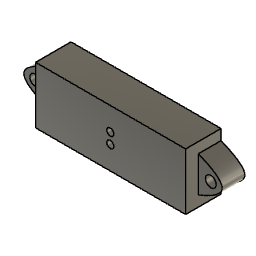
L Distance Sensor Mount (Autodesk Fusion 360 archive; units mm, degrees)
design "Distance Sensor"
Autodesk Fusion 360 part; units mm, degrees
sketch "Sketch2" plane through (0, 0, 0) normal (0, 1, 0) x (1, 0, 0)
  line L0 (0, 0) -> (42.015, 0)
  line L1 (42.015, 0) -> (42.015, -15.89)
  line L2 (42.015, -15.89) -> (0, -15.89)
  line L3 (0, -15.89) -> (0, 0)
  circle A0 centre (45.515, -7.945) radius 1.5
  line L4 (42.015, -7.945) -> (48.69, -7.945)
  spline S0 degree 5 poles (42.015, -12.945) (42.5156, -12.7419) (43.4745, -12.3366) (44.7863, -11.7309) (46.2763, -10.9278) (47.6689, -9.93) (48.5399, -8.9364) (48.8392, -7.945) (48.5399, -6.9536) (47.6689, -5.96) (46.2763, -4.9622) (44.7863, -4.1591) (43.4745, -3.5534) (42.5156, -3.1481) (42.015, -2.945) knots 0 0 0 0 0 0 0.1 0.2 0.3 0.4 0.5 0.6 0.7 0.8 0.9 1 1 1 1 1 1
  line L5 (20.92, -15.89) -> (20.92, 0)
  spline S1 degree 5 poles (-0.175, -12.945) (-0.6756, -12.7419) (-1.6345, -12.3366) (-2.9463, -11.7309) (-4.4363, -10.9278) (-5.8289, -9.93) (-6.6999, -8.9364) (-6.9992, -7.945) (-6.6999, -6.9536) (-5.8289, -5.96) (-4.4363, -4.9622) (-2.9463, -4.1591) (-1.6345, -3.5534) (-0.6756, -3.1481) (-0.175, -2.945) knots 0 0 0 0 0 0 0.1 0.2 0.3 0.4 0.5 0.6 0.7 0.8 0.9 1 1 1 1 1 1
  line L6 (40.2192, -13.6735) -> (43.8108, -12.2165)
  line L7 (43.8108, -3.6735) -> (40.2192, -2.2165)
  line L8 (1.6208, -13.6735) -> (-1.9708, -12.2165)
  line L9 (-1.9708, -3.6735) -> (1.6208, -2.2165)
  circle A1 centre (-3.675, -7.945) radius 1.5
  line L10 (-0.175, -7.945) -> (-6.85, -7.945)
  circle A2 centre (20.92, -9.45) radius 1
  circle A3 centre (20.92, -6.45) radius 1
  line L11 (-0.175, -12.945) -> (0, -13.016)
  line L12 (-0.175, -7.945) -> (0, -7.945)
  line L13 (-0.175, -2.945) -> (0, -2.874)
  dimension "d2" = 15.89
  dimension "d3" = 3
  dimension "d5" = 3.5
  dimension "d6" = 10
  dimension "d7" = 2.945
  dimension "d8" = 15.89
  dimension "d19" = 2
  dimension "d20" = 2
  dimension "d21" = 3
  dimension "d22" = 6.45
  dimension "d25" = 49.19
  dimension "d26" = 42.19
  dimension "d27" = 55.54
  dimension "d29" = 7.945
  constraint horizontal L0
  constraint vertical L1
  constraint horizontal L2
  constraint vertical L3
  constraint coincident L0.start L3.end
  constraint midpoint L1 L4.start
  constraint perpendicular L1 L4
  constraint coincident L1 S0.start
  constraint coincident L1 S0.end
  constraint coincident L2 L5.start
  constraint coincident L0 L5.end
  constraint perpendicular L0 L5
  constraint midpoint S0.start L6
  constraint midpoint S0.end L7
  constraint symmetric A0 L5 A1
  constraint symmetric L4.start L5 L10.start
  constraint symmetric L4.end L5 L10.end
  constraint symmetric S0.start L5 S1.start
  constraint symmetric S0.end L5 S1.end
  constraint symmetric L5 L6.start L8.start
  constraint symmetric L5 L6.end L8.end
  constraint symmetric L5 L7.start L9.start
  constraint symmetric L5 L7.end L9.end
  constraint coincident L5 A2.centre
  constraint coincident L5 A3.centre
  constraint coincident L8 L11.end
  constraint coincident L3 L11.end
  constraint midpoint L3 L12.end
  constraint perpendicular L3 L12
  constraint coincident L9 L13.end
  constraint coincident L3 L13.end
  measures "d2" distance of L0.start L2.end
  measures "d3" diameter of A0
  measures "d5" distance of L1 A0.centre
  measures "d6" distance of S0.start S0.end
  measures "d7" distance of L2 S0.start
  measures "d8" distance of L0.end L1.end
  measures "d19" diameter of A2
  measures "d20" diameter of A3
  measures "d21" distance of A2.centre A3.centre
  measures "d22" distance of L0 A3.centre
  measures "d25" distance of A0.centre A1.centre
  measures "d26" distance of L4.start L10.start
  measures "d27" distance of L4.end L10.end
  measures "d29" distance of L0 A1.centre
extrude "Extrude1" add sketch "Sketch2" along normal blind 6.35 contours L0 L2 L3 L5 A2 A3 | L0 L1 L2 L5 A2 A3 | L3 S1 L9 A1 L10 L12 L13 | L5 A3 | L5 A3 | L3 S1 L8 A1 L10 L11 L12 | L1 A0 L4 S0 | L1 A0 L4 S0 | L5 A2 | L5 A2
extrude "Extrude2" add sketch "Sketch2" against normal blind 3.56 contours L0 L2 L3 L5 A2 A3 | L0 L1 L2 L5 A2 A3 | L5 A3 | L5 A3 | L5 A2 | L5 A2
extrude "Extrude3" cut sketch "Sketch2" against normal blind 25 contours L5 A3 | L5 A3 | L5 A2 | L5 A2
equation "d4 = 6.5 mm"
equation "d5 = d4 - 1.5 mm - d3 / 2"
equation "d7 = ( d8 - d6 ) / 2"
equation "d12 = -9.91 mm + 6.35 mm"
equation "d29 = d2 / 2"

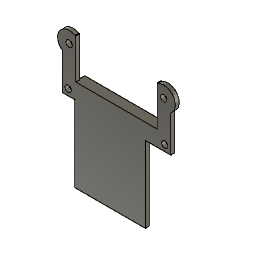
design "hingeMount"
Autodesk Fusion 360 part; units mm, degrees
sketch "Sketch1" plane through (0, 0, 0) normal (0, 0, 1) x (1, 0, 0)
  circle A0 centre (0, 0) radius 1.6
  circle A1 centre (0, 0) radius 3.1
  line L0 (-2.192, 2.192) -> (-8.6341, -4.25)
  line L1 (-2.192, 2.192) -> (4.2881, 2.192) construction
  line L2 (2.192, 2.192) -> (8.6341, -4.25)
  line L3 (2.192, 2.192) -> (10.3664, 2.192) construction
  line L4 (-8.6341, -4.25) -> (8.6341, -4.25)
  dimension "d1" = 3.2
  dimension "d2" = 1.5
  dimension "d3" = 135
  dimension "d4" = 45
  dimension "d5" = 4.25
  constraint coincident A0.centre A1.centre
  constraint horizontal L1
  constraint coincident A1 L0.start
  constraint tangent A1 L0
  constraint horizontal L3
  constraint coincident A1 L2.start
  constraint tangent A1 L2
  constraint horizontal L4
  measures "d1" diameter of A0
  measures "d3" angle of L0 L1
  measures "d4" angle of L2 L3
  measures "d5" distance of A0.centre L4
extrude "Extrude1" add sketch "Sketch1" along normal blind 12.5
extrude "Extrude2" add 1 faces at (-2.878, -4.25, 4.1667) along direction (0, -1, 0) blind 0.8
sketch "Sketch2" plane through (0, -5.05, 0) normal (0, -1, 0) x (1, 0, 0)
  line L0 (-8.6341, 0) -> (8.6341, 0)
  line L1 (8.6341, 0) -> (8.6341, 12.5)
  line L2 (8.6341, 12.5) -> (-8.6341, 12.5)
  line L3 (-8.6341, 12.5) -> (-8.6341, 0)
  line L4 (-8.6341, 12.5) -> (8.6341, 12.5)
  line L5 (8.6341, 12.5) -> (8.6341, -2.5)
  line L6 (8.6341, -2.5) -> (-8.6341, -2.5)
  line L7 (-8.6341, -2.5) -> (-8.6341, 12.5)
  line L8 (-8.6341, 12.5) -> (8.6341, 12.5)
  line L9 (8.6341, 12.5) -> (8.6341, 14)
  line L10 (8.6341, 14) -> (-8.6341, 14)
  line L11 (-8.6341, 14) -> (-8.6341, 12.5)
  dimension "d10" = 15
  dimension "d11" = 1.5
  constraint horizontal L4
  constraint vertical L5
  constraint horizontal L6
  constraint vertical L7
  constraint coincident L2.end L3.start
  constraint horizontal L8
  constraint vertical L9
  constraint horizontal L10
  constraint vertical L11
  measures "d10" distance of L2.end L6.end
  measures "d11" distance of L2.end L10.end
extrude "Extrude3" add sketch "Sketch2" along normal blind 1.5
sketch "Sketch3" plane through (0, -6.55, 0) normal (0, -1, 0) x (1, 0, 0)
  line L0 (8.6341, -2.5) -> (8.6341, 14)
  line L1 (8.6341, 14) -> (-8.6341, 14)
  line L2 (-8.6341, 14) -> (-8.6341, -2.5)
  line L3 (-8.6341, -2.5) -> (8.6341, -2.5)
  line L4 (-21, -2.5) -> (21, -2.5)
  line L5 (21, -2.5) -> (21, 64)
  line L6 (21, 64) -> (-21, 64)
  line L7 (-21, 64) -> (-21, -2.5)
  dimension "d14" = 42
  dimension "d15" = 50
  constraint horizontal L4
  constraint vertical L5
  constraint horizontal L6
  constraint vertical L7
  constraint midpoint L3 L4
  measures "d14" distance of L4.start L4.end
  measures "d15" distance of L1 L6
extrude "Extrude4" add sketch "Sketch3" along normal blind 2
extrude "Extrude5" add 1 faces at (2.878, -5.55, 14) along direction (0, 0, 1) blind 27
sketch "Sketch4" plane through (0, -6.55, 0) normal (0, 1, 0) x (-1, 0, 0)
  line L0 (8.6341, -2.5) -> (21, -2.5)
  line L1 (21, -2.5) -> (21, 64)
  line L2 (21, 64) -> (-21, 64)
  line L3 (-21, 64) -> (-21, -2.5)
  line L4 (-23.9, 59) -> (23.9, 59)
  circle A0 centre (-23.9, 59) radius 5.7801
  circle A1 centre (23.9, 59) radius 5.7801
  line L5 (-23.9, 53.2199) -> (-21, 53.2199)
  line L6 (-21, 53.2199) -> (-21, 40.8199)
  line L7 (-21, 40.8199) -> (-23.9, 40.8199)
  line L8 (-23.9, 40.8199) -> (-23.9, 53.2199)
  line L9 (-23.9, 40.8199) -> (-27.4, 40.8199)
  line L10 (-27.4, 40.8199) -> (-27.4, 53.2199)
  line L11 (-27.4, 53.2199) -> (-23.9, 53.2199)
  line L12 (-23.9, 53.2199) -> (-23.9, 40.8199)
  line L13 (-27.4, 53.2199) -> (-27.4, 54.4)
  line L14 (21, 40.8199) -> (27.4, 40.8199)
  line L15 (27.4, 40.8199) -> (27.4, 53.2199)
  line L16 (27.4, 53.2199) -> (21, 53.2199)
  line L17 (21, 53.2199) -> (21, 40.8199)
  line L18 (27.4, 53.2199) -> (27.4, 54.4)
  line L19 (-27.4, 40.8199) -> (-21, 40.8199)
  line L20 (-21, 40.8199) -> (-21, 35.8199)
  line L21 (-21, 35.8199) -> (-27.4, 35.8199)
  line L22 (-27.4, 35.8199) -> (-27.4, 40.8199)
  line L23 (21, 40.8199) -> (27.4, 40.8199)
  line L24 (27.4, 40.8199) -> (27.4, 35.8199)
  line L25 (27.4, 35.8199) -> (21, 35.8199)
  line L26 (21, 35.8199) -> (21, 40.8199)
  circle A2 centre (-23.9, 59) radius 1.6
  circle A3 centre (23.9, 59) radius 1.6
  line L27 (-27.4, 40.8199) -> (27.4, 40.8199)
  line L28 (27.4, 40.8199) -> (27.4, 43.8699)
  line L29 (27.4, 43.8699) -> (-27.4, 43.8699)
  line L30 (-27.4, 43.8699) -> (-27.4, 40.8199)
  line L31 (-8.6341, 41) -> (8.6341, 41)
  line L32 (8.6341, 41) -> (8.6341, -2.5)
  line L33 (-21, -2.5) -> (-8.6341, -2.5)
  line L34 (-8.6341, -2.5) -> (-8.6341, 41)
  point P0 (0, 59)
  point P1 (-23.9, 53.2199)
  dimension "d21" = 47.8
  dimension "d22" = 5
  dimension "d23" = 21
  dimension "d26" = 12.4
  dimension "d27" = 2.9
  dimension "d28" = 3.5
  dimension "d29" = 6.4
  dimension "d31" = 12.4
  dimension "d32" = 5
  dimension "d33" = 5
  dimension "d34" = 3.2
  dimension "d35" = 3.2
  dimension "d36" = 3.05
  constraint horizontal L4
  constraint midpoint L4 P0
  constraint coincident L4.start A0.centre
  constraint coincident L2.end A0
  constraint coincident L4.end A1.centre
  constraint coincident L1.end A1
  constraint coincident A0 P1
  constraint horizontal L5
  constraint vertical L6
  constraint horizontal L7
  constraint vertical L8
  constraint coincident L3 L6.end
  constraint coincident P1 L5.start
  constraint horizontal L9
  constraint vertical L10
  constraint horizontal L11
  constraint vertical L12
  constraint coincident A0 L13.end
  constraint perpendicular L11 L13
  constraint horizontal L14
  constraint vertical L15
  constraint horizontal L16
  constraint vertical L17
  constraint coincident L1 L14.start
  constraint coincident A1 L18.end
  constraint perpendicular L16 L18
  constraint tangent A1 L16
  constraint horizontal L19
  constraint vertical L20
  constraint horizontal L21
  constraint vertical L22
  constraint horizontal L23
  constraint vertical L24
  constraint horizontal L25
  constraint vertical L26
  constraint coincident L14.end L15.start
  constraint concentric A0 A2
  constraint concentric A1 A3
  constraint horizontal L27
  constraint vertical L28
  constraint horizontal L29
  constraint vertical L30
  constraint coincident L15 L28.end
  measures "d21" distance of L4.start L4.end
  measures "d22" distance of L2 L4
  measures "d23" distance of L3 P0
  measures "d26" distance of P1 L7.end
  measures "d27" distance of L6.end L7.end
  measures "d28" distance of L7.end L9.end
  measures "d29" distance of L14.start L14.end
  measures "d31" distance of L14.end L15.end
  measures "d32" distance of L9.end L21.end
  measures "d33" distance of L14.start L25.end
  measures "d34" diameter of A2
  measures "d35" diameter of A3
  measures "d36" distance of L9.end L29.end
extrude "Extrude6" add sketch "Sketch4" against normal blind 2 contours L1 L14 L23 L24 L25 L26 L27 | L1 L14 L15 L17 L23 L27 L28 L29 | L3 L6 L7 L8 L12 L19 L27 L29 | L3 L7 L9 L19 L20 L21 L22 L27 | L1 L15 L16 L17 L29 | L3 L5 L6 L8 L12 L29 | L8 L9 L10 L12 L19 L27 L29 L30 | L1 A1 L16 | L3 A0 L5 | L8 L10 L11 L12 L29 | L1 A1 | A1 L16 L18 | L3 A0 | A0 L11 L13
extrude "Extrude7" add sketch "Sketch4" along normal blind 3 contours L1 L3 L6 L17 L27 L29 L31 L32 L34 | L27 L31 L32 L34
chamfer "Chamfer1" distance 1.5 angle 45 4 edges at (-14.817, -6.55, 40.8199) (-8.6341, -6.55, 19.1599) (8.6341, -6.55, 19.1599) (14.817, -6.55, 40.8199)
sketch "Sketch5" plane through (0, -6.55, 0) normal (0, 1, 0) x (-1, 0, 0)
  line L0 (10.1341, 39.3199) -> (10.1341, -2.5)
  line L1 (10.1341, -2.5) -> (21, -2.5)
  line L2 (21, -2.5) -> (21, 35.8199)
  line L3 (21, 35.8199) -> (27.4, 35.8199)
  line L4 (27.4, 35.8199) -> (27.4, 54.4)
  arc A0 (27.4, 54.4) -> (21, 64) centre (23.9, 59) ccw
  line L5 (21, 64) -> (-21, 64)
  arc A1 (-21, 64) -> (-27.4, 54.4) centre (-23.9, 59) ccw
  line L6 (-27.4, 54.4) -> (-27.4, 35.8199)
  line L7 (-27.4, 35.8199) -> (-21, 35.8199)
  line L8 (-21, 35.8199) -> (-21, -2.5)
  line L9 (-21, -2.5) -> (-10.1341, -2.5)
  line L10 (-10.1341, -2.5) -> (-10.1341, 39.3199)
  line L11 (-10.1341, 39.3199) -> (-21, 39.3199)
  line L12 (-21, 43.8699) -> (21, 43.8699)
  line L13 (21, 39.3199) -> (10.1341, 39.3199)
  circle A2 centre (23.9, 59) radius 1.6
  circle A3 centre (-23.9, 59) radius 1.6
  line L14 (-21, 43.8699) -> (21, 43.8699)
  line L15 (-20.5, 64) -> (20.5, 64)
  line L16 (20.5, 64) -> (20.5, 43.8699)
  line L17 (20.5, 43.8699) -> (-20.5, 43.8699)
  line L18 (-20.5, 43.8699) -> (-20.5, 64)
  line L19 (-21, 39.3199) -> (-21, 43.8699)
  line L20 (21, 43.8699) -> (21, 39.3199)
  dimension "d40" = 41
  constraint horizontal L15
  constraint vertical L16
  constraint horizontal L17
  constraint vertical L18
  constraint midpoint L5 L15
  constraint midpoint L12 L17
  measures "d40" distance of L15.start L15.end
extrude "Extrude8" cut sketch "Sketch5" against normal blind 2 contours L5 L12 L14 L15 L16 L17 L18
sketch "Sketch6" plane through (0, -8.55, 0) normal (0, -1, 0) x (1, 0, 0)
  line L0 (20.5, 64) -> (20.5, 43.8699)
  line L1 (20.5, 43.8699) -> (-20.5, 43.8699)
  line L2 (-20.5, 43.8699) -> (-20.5, 64)
  line L3 (-20.5, 64) -> (-21, 64)
  arc A0 (-21, 64) -> (-27.4, 54.4) centre (-23.9, 59) ccw
  line L4 (-27.4, 54.4) -> (-27.4, 35.8199)
  line L5 (-27.4, 35.8199) -> (-21, 35.8199)
  line L6 (-21, 35.8199) -> (-21, -2.5)
  line L7 (-21, -2.5) -> (21, -2.5)
  line L8 (21, -2.5) -> (21, 35.8199)
  line L9 (21, 35.8199) -> (27.4, 35.8199)
  line L10 (27.4, 35.8199) -> (27.4, 54.4)
  arc A1 (27.4, 54.4) -> (21, 64) centre (23.9, 59) ccw
  line L11 (21, 64) -> (20.5, 64)
  circle A2 centre (23.9, 59) radius 1.6
  circle A3 centre (-23.9, 59) radius 1.6
  circle A4 centre (-24.4, 39) radius 1.6
  circle A5 centre (24.4, 39) radius 1.6
  line L12 (27.4, 43.8636) -> (-27.4, 43.8636)
  line L13 (-27.4, 43.8636) -> (-27.4, 23.8636)
  line L14 (-27.4, 23.8636) -> (27.4, 23.8636)
  line L15 (27.4, 23.8636) -> (27.4, 43.8636)
  dimension "d43" = 3.2
  dimension "d45" = 3.2
  dimension "d46" = 20
  dimension "d60" = 3
  dimension "d61" = 20
  dimension "d62" = 3
  dimension "d63" = 20
  constraint horizontal L12
  constraint vertical L13
  constraint horizontal L14
  constraint vertical L15
  constraint coincident L10 L12.start
  measures "d43" diameter of A4
  measures "d45" diameter of A5
  measures "d46" distance of L12.start L14.end
  measures "d60" distance of A4.centre L13
  measures "d61" vertical distance of A0.centre A4.centre
  measures "d62" distance of A5.centre L15
  measures "d63" vertical distance of A1.centre A5.centre
extrude "Extrude9" cut sketch "Sketch6" against normal blind 2 contours A4 | A5
extrude "Extrude10" add sketch "Sketch6" along normal blind 1.25 contours L4 L5 L6 L8 L9 L10 L12 L13 L14 L15 | L8 L9 L14 L15 | L5 L6 L13 L14
ref_plane "WorkPlane1" through (-21, -8.175, 39.1318) normal (-1, 0, 0) x (0, 0, -1)
sketch "Sketch7" plane through (-21, 0, 0) normal (-1, 0, 0) x (0, -1, 0)
  circle A0 centre (13.225, 30.398) radius 1.625
  line L0 (9.8, 43.8636) -> (9.8, 23.8636)
  circle A1 centre (13.225, 30.398) radius 3.125
  line L1 (13.225, 33.523) -> (9.8, 33.523)
  line L2 (9.8, 23.8636) -> (15.1177, 27.9114)
  dimension "d52" = 3.25
  dimension "d53" = 3.425
  dimension "d54" = 1.5
  constraint coincident A1 L1.start
  constraint coincident L0 L1.end
  constraint tangent A1 L1
  constraint perpendicular L0 L1
  constraint coincident L0.end L2.start
  constraint coincident A1 L2.end
  constraint tangent A1 L2
  measures "d52" diameter of A0
  measures "d53" distance of A0.centre L0
extrude "Extrude11" add sketch "Sketch7" against normal blind 42
sketch "Sketch8" plane through (0, 0, 43.8699) normal (0, 0, 1) x (-1, 0, 0)
  line L0 (-20.5, 6.55) -> (-21, 6.55)
  line L1 (-21, 6.55) -> (-21, 3.55)
  line L2 (-21, 3.55) -> (21, 3.55)
  line L3 (21, 3.55) -> (21, 6.55)
  line L4 (21, 6.55) -> (20.5, 6.55)
  line L5 (20.5, 6.55) -> (20.5, 8.55)
  line L6 (20.5, 8.55) -> (-20.5, 8.55)
  line L7 (-20.5, 8.55) -> (-20.5, 6.55)
  line L8 (16.5, 9.8) -> (-16.5, 9.8)
  line L9 (-16.5, 9.8) -> (-16.5, 17.8932)
  line L10 (-16.5, 17.8932) -> (16.5, 17.8932)
  line L11 (16.5, 17.8932) -> (16.5, 9.8)
  dimension "d57" = 33
  constraint horizontal L8
  constraint vertical L9
  constraint horizontal L10
  constraint vertical L11
  measures "d57" distance of L8.start L8.end
extrude "Extrude12" cut sketch "Sketch8" against normal blind 20 contours L8 L9 L10 L11
sketch "Sketch9" plane through (0, 0, -2.5) normal (0, 0, -1) x (1, 0, 0)
  line L0 (-8.6341, 5.05) -> (8.6341, 5.05)
  line L1 (8.6341, 5.05) -> (10.1341, 6.55)
  line L2 (10.1341, 6.55) -> (21, 6.55)
  line L3 (21, 6.55) -> (21, 8.55)
  line L4 (21, 8.55) -> (-21, 8.55)
  line L5 (-21, 8.55) -> (-21, 6.55)
  line L6 (-21, 6.55) -> (-10.1341, 6.55)
  line L7 (-10.1341, 6.55) -> (-8.6341, 5.05)
  line L8 (-33.0946, 8.55) -> (32.2741, 8.55)
  line L9 (32.2741, 8.55) -> (32.2741, 20.9691)
  line L10 (32.2741, 20.9691) -> (-33.0946, 20.9691)
  line L11 (-33.0946, 20.9691) -> (-33.0946, 8.55)
  constraint horizontal L8
  constraint vertical L9
  constraint horizontal L10
  constraint vertical L11
extrude "Extrude13" cut sketch "Sketch9" against normal blind 56 contours L4 L8 L9 L10 L11
extrude "Extrude14" cut 1 faces at (25.2667, -7.8833, 35.8199) along direction (0, 0, 1) blind 0.1
extrude "Extrude15" cut 1 faces at (-25.2667, -7.2167, 35.8199) along direction (0, 0, 1) blind 0.1
extrude "Extrude16" cut 1 faces at (21, -7.8833, 10.3066) along direction (-1, 0, 0) blind 4.5
extrude "Extrude17" cut 1 faces at (16.5, -7.8833, 10.3066) along direction (-1, 0, 0) blind 1.9
chamfer "Chamfer2" [suppressed]
equation "d5 = 1.6 mm + 1.5 mm + 1.15 mm"
equation "d53 = 1.8 mm + ( 3.25 / 2 ) * 1 mm"

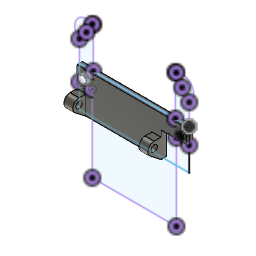
design "cataMount"
Autodesk Fusion 360 part; units mm, degrees
sketch "Sketch1" plane through (0, 0, 0) normal (0, 0, 1) x (1, 0, 0)
  circle A0 centre (0, 0) radius 1.6
  circle A1 centre (0, 0) radius 3.1
  line L0 (-2.192, 2.192) -> (-8.6341, -4.25)
  line L1 (-2.192, 2.192) -> (4.2881, 2.192) construction
  line L2 (2.192, 2.192) -> (8.6341, -4.25)
  line L3 (2.192, 2.192) -> (10.3664, 2.192) construction
  line L4 (-8.6341, -4.25) -> (8.6341, -4.25)
  dimension "d1" = 3.2
  dimension "d2" = 1.5
  dimension "d3" = 135
  dimension "d4" = 45
  dimension "d5" = 4.25
  constraint coincident A0.centre A1.centre
  constraint horizontal L1
  constraint coincident A1 L0.start
  constraint tangent A1 L0
  constraint horizontal L3
  constraint coincident A1 L2.start
  constraint tangent A1 L2
  constraint horizontal L4
  measures "d1" diameter of A0
  measures "d3" angle of L0 L1
  measures "d4" angle of L2 L3
  measures "d5" distance of A0.centre L4
extrude "Extrude1" add sketch "Sketch1" along normal blind 12.5
extrude "Extrude2" add 1 faces at (-2.878, -4.25, 4.1667) along direction (0, -1, 0) blind 0.8
sketch "Sketch2" plane through (0, -5.05, 0) normal (0, -1, 0) x (1, 0, 0)
  line L0 (-8.6341, 0) -> (8.6341, 0)
  line L1 (8.6341, 0) -> (8.6341, 12.5)
  line L2 (8.6341, 12.5) -> (-8.6341, 12.5)
  line L3 (-8.6341, 12.5) -> (-8.6341, 0)
  line L4 (-8.6341, 12.5) -> (8.6341, 12.5)
  line L5 (8.6341, 12.5) -> (8.6341, -2.5)
  line L6 (8.6341, -2.5) -> (-8.6341, -2.5)
  line L7 (-8.6341, -2.5) -> (-8.6341, 12.5)
  line L8 (-8.6341, 12.5) -> (8.6341, 12.5)
  line L9 (8.6341, 12.5) -> (8.6341, 14)
  line L10 (8.6341, 14) -> (-8.6341, 14)
  line L11 (-8.6341, 14) -> (-8.6341, 12.5)
  dimension "d10" = 15
  dimension "d11" = 1.5
  constraint horizontal L4
  constraint vertical L5
  constraint horizontal L6
  constraint vertical L7
  constraint coincident L2.end L3.start
  constraint horizontal L8
  constraint vertical L9
  constraint horizontal L10
  constraint vertical L11
  measures "d10" distance of L2.end L6.end
  measures "d11" distance of L2.end L10.end
extrude "Extrude3" add sketch "Sketch2" along normal blind 1.5
sketch "Sketch3" plane through (0, -6.55, 0) normal (0, -1, 0) x (1, 0, 0)
  line L0 (8.6341, -2.5) -> (8.6341, 14)
  line L1 (8.6341, 14) -> (-8.6341, 14)
  line L2 (-8.6341, 14) -> (-8.6341, -2.5)
  line L3 (-8.6341, -2.5) -> (8.6341, -2.5)
  line L4 (-21, -2.5) -> (21, -2.5)
  line L5 (21, -2.5) -> (21, 64)
  line L6 (21, 64) -> (-21, 64)
  line L7 (-21, 64) -> (-21, -2.5)
  dimension "d14" = 42
  dimension "d15" = 50
  constraint horizontal L4
  constraint vertical L5
  constraint horizontal L6
  constraint vertical L7
  constraint midpoint L3 L4
  measures "d14" distance of L4.start L4.end
  measures "d15" distance of L1 L6
extrude "Extrude4" add sketch "Sketch3" along normal blind 2
extrude "Extrude5" add 1 faces at (2.878, -5.55, 14) along direction (0, 0, 1) blind 27
sketch "Sketch4" plane through (0, -6.55, 0) normal (0, 1, 0) x (-1, 0, 0)
  line L0 (8.6341, -2.5) -> (21, -2.5)
  line L1 (21, -2.5) -> (21, 64)
  line L2 (21, 64) -> (-21, 64)
  line L3 (-21, 64) -> (-21, -2.5)
  line L4 (-23.9, 59) -> (23.9, 59)
  circle A0 centre (-23.9, 59) radius 5.7801
  circle A1 centre (23.9, 59) radius 5.7801
  line L5 (-23.9, 53.2199) -> (-21, 53.2199)
  line L6 (-21, 53.2199) -> (-21, 40.8199)
  line L7 (-21, 40.8199) -> (-23.9, 40.8199)
  line L8 (-23.9, 40.8199) -> (-23.9, 53.2199)
  line L9 (-23.9, 40.8199) -> (-27.4, 40.8199)
  line L10 (-27.4, 40.8199) -> (-27.4, 53.2199)
  line L11 (-27.4, 53.2199) -> (-23.9, 53.2199)
  line L12 (-23.9, 53.2199) -> (-23.9, 40.8199)
  line L13 (-27.4, 53.2199) -> (-27.4, 54.4)
  line L14 (21, 40.8199) -> (27.4, 40.8199)
  line L15 (27.4, 40.8199) -> (27.4, 53.2199)
  line L16 (27.4, 53.2199) -> (21, 53.2199)
  line L17 (21, 53.2199) -> (21, 40.8199)
  line L18 (27.4, 53.2199) -> (27.4, 54.4)
  line L19 (-27.4, 40.8199) -> (-21, 40.8199)
  line L20 (-21, 40.8199) -> (-21, 35.8199)
  line L21 (-21, 35.8199) -> (-27.4, 35.8199)
  line L22 (-27.4, 35.8199) -> (-27.4, 40.8199)
  line L23 (21, 40.8199) -> (27.4, 40.8199)
  line L24 (27.4, 40.8199) -> (27.4, 35.8199)
  line L25 (27.4, 35.8199) -> (21, 35.8199)
  line L26 (21, 35.8199) -> (21, 40.8199)
  circle A2 centre (-23.9, 59) radius 1.6
  circle A3 centre (23.9, 59) radius 1.6
  line L27 (-27.4, 40.8199) -> (27.4, 40.8199)
  line L28 (27.4, 40.8199) -> (27.4, 43.8699)
  line L29 (27.4, 43.8699) -> (-27.4, 43.8699)
  line L30 (-27.4, 43.8699) -> (-27.4, 40.8199)
  line L31 (-8.6341, 41) -> (8.6341, 41)
  line L32 (8.6341, 41) -> (8.6341, -2.5)
  line L33 (-21, -2.5) -> (-8.6341, -2.5)
  line L34 (-8.6341, -2.5) -> (-8.6341, 41)
  point P0 (0, 59)
  point P1 (-23.9, 53.2199)
  dimension "d21" = 47.8
  dimension "d22" = 5
  dimension "d23" = 21
  dimension "d26" = 12.4
  dimension "d27" = 2.9
  dimension "d28" = 3.5
  dimension "d29" = 6.4
  dimension "d31" = 12.4
  dimension "d32" = 5
  dimension "d33" = 5
  dimension "d34" = 3.2
  dimension "d35" = 3.2
  dimension "d36" = 3.05
  constraint horizontal L4
  constraint midpoint L4 P0
  constraint coincident L4.start A0.centre
  constraint coincident L2.end A0
  constraint coincident L4.end A1.centre
  constraint coincident L1.end A1
  constraint coincident A0 P1
  constraint horizontal L5
  constraint vertical L6
  constraint horizontal L7
  constraint vertical L8
  constraint coincident L3 L6.end
  constraint coincident P1 L5.start
  constraint horizontal L9
  constraint vertical L10
  constraint horizontal L11
  constraint vertical L12
  constraint coincident A0 L13.end
  constraint perpendicular L11 L13
  constraint horizontal L14
  constraint vertical L15
  constraint horizontal L16
  constraint vertical L17
  constraint coincident L1 L14.start
  constraint coincident A1 L18.end
  constraint perpendicular L16 L18
  constraint tangent A1 L16
  constraint horizontal L19
  constraint vertical L20
  constraint horizontal L21
  constraint vertical L22
  constraint horizontal L23
  constraint vertical L24
  constraint horizontal L25
  constraint vertical L26
  constraint coincident L14.end L15.start
  constraint concentric A0 A2
  constraint concentric A1 A3
  constraint horizontal L27
  constraint vertical L28
  constraint horizontal L29
  constraint vertical L30
  constraint coincident L15 L28.end
  measures "d21" distance of L4.start L4.end
  measures "d22" distance of L2 L4
  measures "d23" distance of L3 P0
  measures "d26" distance of P1 L7.end
  measures "d27" distance of L6.end L7.end
  measures "d28" distance of L7.end L9.end
  measures "d29" distance of L14.start L14.end
  measures "d31" distance of L14.end L15.end
  measures "d32" distance of L9.end L21.end
  measures "d33" distance of L14.start L25.end
  measures "d34" diameter of A2
  measures "d35" diameter of A3
  measures "d36" distance of L9.end L29.end
extrude "Extrude6" add sketch "Sketch4" against normal blind 2 contours L1 L14 L23 L24 L25 L26 L27 | L1 L14 L15 L17 L23 L27 L28 L29 | L3 L6 L7 L8 L12 L19 L27 L29 | L3 L7 L9 L19 L20 L21 L22 L27 | L1 L15 L16 L17 L29 | L3 L5 L6 L8 L12 L29 | L8 L9 L10 L12 L19 L27 L29 L30 | L1 A1 L16 | L3 A0 L5 | L8 L10 L11 L12 L29 | L1 A1 | A1 L16 L18 | L3 A0 | A0 L11 L13
extrude "Extrude7" add sketch "Sketch4" along normal blind 3 contours L1 L3 L6 L17 L27 L29 L31 L32 L34 | L27 L31 L32 L34
chamfer "Chamfer1" distance 1.5 angle 45 4 edges at (-14.817, -6.55, 40.8199) (-8.6341, -6.55, 19.1599) (8.6341, -6.55, 19.1599) (14.817, -6.55, 40.8199)
sketch "Sketch5" plane through (0, -6.55, 0) normal (0, 1, 0) x (-1, 0, 0)
  line L0 (10.1341, 39.3199) -> (10.1341, -2.5)
  line L1 (10.1341, -2.5) -> (21, -2.5)
  line L2 (21, -2.5) -> (21, 35.8199)
  line L3 (21, 35.8199) -> (27.4, 35.8199)
  line L4 (27.4, 35.8199) -> (27.4, 54.4)
  arc A0 (27.4, 54.4) -> (21, 64) centre (23.9, 59) ccw
  line L5 (21, 64) -> (-21, 64)
  arc A1 (-21, 64) -> (-27.4, 54.4) centre (-23.9, 59) ccw
  line L6 (-27.4, 54.4) -> (-27.4, 35.8199)
  line L7 (-27.4, 35.8199) -> (-21, 35.8199)
  line L8 (-21, 35.8199) -> (-21, -2.5)
  line L9 (-21, -2.5) -> (-10.1341, -2.5)
  line L10 (-10.1341, -2.5) -> (-10.1341, 39.3199)
  line L11 (-10.1341, 39.3199) -> (-21, 39.3199)
  line L12 (-21, 43.8699) -> (21, 43.8699)
  line L13 (21, 39.3199) -> (10.1341, 39.3199)
  circle A2 centre (23.9, 59) radius 1.6
  circle A3 centre (-23.9, 59) radius 1.6
  line L14 (-21, 43.8699) -> (21, 43.8699)
  line L15 (-20.5, 64) -> (20.5, 64)
  line L16 (20.5, 64) -> (20.5, 43.8699)
  line L17 (20.5, 43.8699) -> (-20.5, 43.8699)
  line L18 (-20.5, 43.8699) -> (-20.5, 64)
  line L19 (-21, 39.3199) -> (-21, 43.8699)
  line L20 (21, 43.8699) -> (21, 39.3199)
  dimension "d40" = 41
  constraint horizontal L15
  constraint vertical L16
  constraint horizontal L17
  constraint vertical L18
  constraint midpoint L5 L15
  constraint midpoint L12 L17
  measures "d40" distance of L15.start L15.end
extrude "Extrude8" cut sketch "Sketch5" against normal blind 2 contours L5 L12 L14 L15 L16 L17 L18
sketch "Sketch6" plane through (0, -8.55, 0) normal (0, -1, 0) x (1, 0, 0)
  line L0 (20.5, 64) -> (20.5, 43.8699)
  line L1 (20.5, 43.8699) -> (-20.5, 43.8699)
  line L2 (-20.5, 43.8699) -> (-20.5, 64)
  line L3 (-20.5, 64) -> (-21, 64)
  arc A0 (-21, 64) -> (-27.4, 54.4) centre (-23.9, 59) ccw
  line L4 (-27.4, 54.4) -> (-27.4, 35.8199)
  line L5 (-27.4, 35.8199) -> (-21, 35.8199)
  line L6 (-21, 35.8199) -> (-21, -2.5)
  line L7 (-21, -2.5) -> (21, -2.5)
  line L8 (21, -2.5) -> (21, 35.8199)
  line L9 (21, 35.8199) -> (27.4, 35.8199)
  line L10 (27.4, 35.8199) -> (27.4, 54.4)
  arc A1 (27.4, 54.4) -> (21, 64) centre (23.9, 59) ccw
  line L11 (21, 64) -> (20.5, 64)
  circle A2 centre (23.9, 59) radius 1.6
  circle A3 centre (-23.9, 59) radius 1.6
  circle A4 centre (-24.4, 39) radius 1.6
  circle A5 centre (24.4, 39) radius 1.6
  line L12 (27.4, 43.8636) -> (-27.4, 43.8636)
  line L13 (-27.4, 43.8636) -> (-27.4, 23.8636)
  line L14 (-27.4, 23.8636) -> (27.4, 23.8636)
  line L15 (27.4, 23.8636) -> (27.4, 43.8636)
  dimension "d43" = 3.2
  dimension "d45" = 3.2
  dimension "d46" = 20
  dimension "d60" = 3
  dimension "d61" = 20
  dimension "d62" = 3
  dimension "d63" = 20
  constraint horizontal L12
  constraint vertical L13
  constraint horizontal L14
  constraint vertical L15
  constraint coincident L10 L12.start
  measures "d43" diameter of A4
  measures "d45" diameter of A5
  measures "d46" distance of L12.start L14.end
  measures "d60" distance of A4.centre L13
  measures "d61" vertical distance of A0.centre A4.centre
  measures "d62" distance of A5.centre L15
  measures "d63" vertical distance of A1.centre A5.centre
extrude "Extrude9" cut sketch "Sketch6" against normal blind 2 contours A4 | A5
extrude "Extrude10" add sketch "Sketch6" along normal blind 1.25 contours L4 L5 L6 L8 L9 L10 L12 L13 L14 L15 | L8 L9 L14 L15 | L5 L6 L13 L14
ref_plane "WorkPlane1" through (-21, -8.175, 39.1318) normal (-1, 0, 0) x (0, 0, -1)
sketch "Sketch7" plane through (-21, 0, 0) normal (-1, 0, 0) x (0, -1, 0)
  circle A0 centre (13.225, 30.398) radius 1.625
  line L0 (9.8, 43.8636) -> (9.8, 23.8636)
  circle A1 centre (13.225, 30.398) radius 3.125
  line L1 (13.225, 33.523) -> (9.8, 33.523)
  line L2 (9.8, 23.8636) -> (15.1177, 27.9114)
  dimension "d52" = 3.25
  dimension "d53" = 3.425
  dimension "d54" = 1.5
  constraint coincident A1 L1.start
  constraint coincident L0 L1.end
  constraint tangent A1 L1
  constraint perpendicular L0 L1
  constraint coincident L0.end L2.start
  constraint coincident A1 L2.end
  constraint tangent A1 L2
  measures "d52" diameter of A0
  measures "d53" distance of A0.centre L0
extrude "Extrude11" add sketch "Sketch7" along normal blind -35.6 and the other way blind -6.4
sketch "Sketch8" plane through (0, 0, 43.8699) normal (0, 0, 1) x (-1, 0, 0)
  line L0 (-20.5, 6.55) -> (-21, 6.55)
  line L1 (-21, 6.55) -> (-21, 3.55)
  line L2 (-21, 3.55) -> (21, 3.55)
  line L3 (21, 3.55) -> (21, 6.55)
  line L4 (21, 6.55) -> (20.5, 6.55)
  line L5 (20.5, 6.55) -> (20.5, 8.55)
  line L6 (20.5, 8.55) -> (-20.5, 8.55)
  line L7 (-20.5, 8.55) -> (-20.5, 6.55)
  line L8 (22.9, 9.8) -> (-10.1, 9.8)
  line L9 (-10.1, 9.8) -> (-10.1, 17.8932)
  line L10 (-10.1, 17.8932) -> (22.9, 17.8932)
  line L11 (22.9, 17.8932) -> (22.9, 9.8)
  line L12 (27.4, 6.55) -> (27.4, 8.55)
  line L13 (27.4, 9.8) -> (-14.6, 9.8)
  dimension "d57" = 33
  dimension "d74" = 4.5
  dimension "d75" = 42
  constraint horizontal L8
  constraint vertical L9
  constraint horizontal L10
  constraint vertical L11
  measures "d57" distance of L8.start L8.end
  measures "d74" distance of L11 L12
  measures "d75" distance of L13.start L13.end
extrude "Extrude12" cut sketch "Sketch8" against normal blind 20 contours L8 L9 L10 L11 L13
sketch "Sketch9" plane through (0, 0, -2.5) normal (0, 0, -1) x (1, 0, 0)
  line L0 (-8.6341, 5.05) -> (8.6341, 5.05)
  line L1 (8.6341, 5.05) -> (10.1341, 6.55)
  line L2 (10.1341, 6.55) -> (21, 6.55)
  line L3 (21, 6.55) -> (21, 8.55)
  line L4 (21, 8.55) -> (-21, 8.55)
  line L5 (-21, 8.55) -> (-21, 6.55)
  line L6 (-21, 6.55) -> (-10.1341, 6.55)
  line L7 (-10.1341, 6.55) -> (-8.6341, 5.05)
  line L8 (-33.523, 8.55) -> (40.0939, 8.55)
  line L9 (40.0939, 8.55) -> (40.0939, -4.9004)
  line L10 (40.0939, -4.9004) -> (-33.523, -4.9004)
  line L11 (-33.523, -4.9004) -> (-33.523, 8.55)
  constraint horizontal L8
  constraint vertical L9
  constraint horizontal L10
  constraint vertical L11
extrude "Extrude13" cut sketch "Sketch9" against normal blind 75
extrude "Extrude14" add 1 faces at (-7.6927, -8.55, 28.6086) along direction (0, 1, 0) blind 1.5
sketch "Sketch10" plane through (27.4, 0, 0) normal (1, 0, 0) x (0, 1, 0)
  line L0 (-7.05, 43.8636) -> (-9.8, 43.8636)
  line L1 (-9.8, 43.8636) -> (-9.8, 23.8636)
  line L2 (-9.8, 23.8636) -> (-7.05, 23.8636)
  line L3 (-7.05, 23.8636) -> (-7.05, 43.8636)
  line L4 (-9.8, 36.0032) -> (-7.05, 36.0032)
  line L5 (-7.05, 36.0032) -> (-7.05, 23.8636)
  line L6 (-7.05, 23.8636) -> (-9.8, 23.8636)
  line L7 (-9.8, 23.8636) -> (-9.8, 36.0032)
  constraint horizontal L4
  constraint vertical L5
  constraint horizontal L6
  constraint vertical L7
  constraint coincident L2.end L3.start
  constraint coincident L1 L4.start
extrude "Extrude15" cut sketch "Sketch10" against normal blind 6.4 contours L1 L2 L3 L4 L5 L6 L7
extrude "Extrude16" cut 1 faces at (25.2667, -8.8833, 36.0032) along direction (0, 0, 1) blind 0.6
extrude "Extrude17" cut 1 faces at (21, -8.8833, 32.3567) along direction (-1, 0, 0) blind 6.4
equation "d5 = 1.6 mm + 1.5 mm + 1.15 mm"
equation "d53 = 1.8 mm + ( 3.25 / 2 ) * 1 mm"
equation "d55 = -42 mm + 6.4 mm"
equation "d74 = ( d75 - d57 ) / 2"

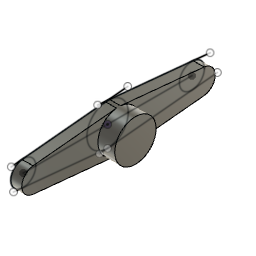
design "motorAttachment"
Autodesk Fusion 360 part; units mm, degrees
sketch "Sketch1" plane through (0, 0, 0) normal (1, 0, 0) x (0, 1, 0)
  circle A0 centre (0, 0) radius 4.15
  line L0 (-16.945, 0) -> (16.945, 0)
  circle A1 centre (16.945, 0) radius 2.5
  circle A2 centre (-16.945, 0) radius 2.5
  line L1 (-19.3593, 2.2757) -> (4.0461, 4.5657)
  line L2 (-18.9011, -2.3206) -> (0.0097, -4.1708)
  line L3 (-1.6323, -4.3295) -> (22.0593, -2.0116)
  line L4 (-1.9945, 4.365) -> (20.605, 2.1539)
  dimension "d1" = 8.3
  dimension "d2" = 33.89
  dimension "d3" = 5
  dimension "d4" = 5
  constraint coincident A0.centre origin
  constraint horizontal L0
  constraint midpoint A0.centre L0
  constraint coincident L0.end A1.centre
  constraint coincident L0.start A2.centre
  constraint tangent A0 L1
  constraint tangent A2 L1
  constraint tangent A2 L2
  constraint tangent A0 L2
  constraint tangent A0 L4
  constraint tangent A1 L4
  constraint tangent A1 L3
  constraint tangent A0 L3
  measures "d1" diameter of A0
  measures "d2" distance of L0.start L0.end
  measures "d3" diameter of A1
  measures "d4" diameter of A2
extrude "Extrude1" add sketch "Sketch1" along normal blind 5.6 contours A0 L0 | A0 L0
extrude "Extrude2" add sketch "Sketch1" along normal blind 2.2 contours A0 L0 A1 L3 | A0 L0 A1 L4 | A0 L0 A2 L1 | A0 L0 A2 L2 | A1 | A2
